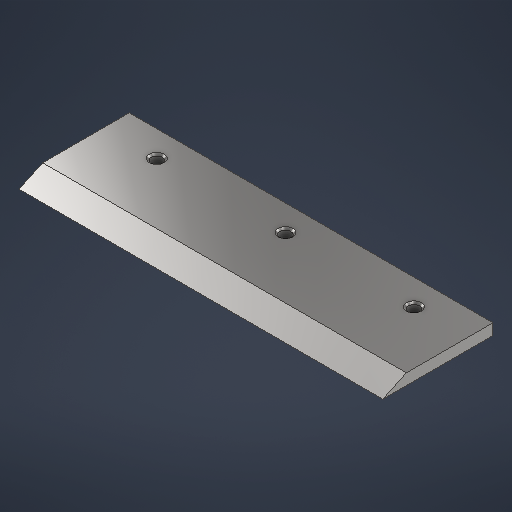
# Autodesk Inventor part: Knife
Saved by Autodesk Inventor 2027 (Build 310192000, 192)
## iProperties
Created: 2026-04-01
Part Number: Knife
Material: Ocel, uhlík
Document SubType Name: Modeling
Designer: zak
Density: 7.85 g/cm^3
Appearance: Pololeštěná
Author: zak
Autodesk Inventor part; units mm, degrees
ref_plane "YZ Plane" through (0, 0, 0) normal (1, 0, 0) x (0, 1, 0)
ref_plane "XZ Plane" through (0, 0, 0) normal (0, 1, 0) x (-1, 0, 0)
ref_plane "XY Plane" through (0, 0, 0) normal (0, 0, 1) x (1, 0, 0)
sketch "Náčrt1" plane through (0, 0, 0) normal (1, 0, 0) x (0, 1, 0)
  line L0 (1.5, 15) -> (-1.5, 15)
  line L1 (-1.5, 15) -> (-1.5, -15)
  line L2 (-1.5, -15) -> (1.5, -15)
  line L3 (1.5, -15) -> (1.5, 15)
  line L4 (1.5, 15) -> (-1.5, -15) construction
  line L5 (-1.5, 15) -> (1.5, -15) construction
  line L6 (-1.5, 15) -> (1.5, 8.5665)
  point P0 (0, 0)
  dimension "d0" = 3
  dimension "d1" = 30
  dimension "d2" = 25
  constraints: 14 end point, 2 midpoint, 2 parallel, 1 horizontal, 1 perpendicular, 1 point on line
  measures "d0" distance between parallel lines of L1 L3
  measures "d1" distance between parallel lines of L0 L2
  measures "d2" angle of L1 L6
extrude "Vysunutí1" add sketch "Náčrt1" along normal mid plane 99 contours L6 L3 L2 L1
sketch "Náčrt2" plane through (-49.5, -1.5, -15) normal (0, -1, 0) x (1, 0, 0)
  circle A0 centre (84.5, 7) radius 1.5
  circle A1 centre (49.5, 7) radius 1.5
  circle A2 centre (14.5, 7) radius 1.5
  line L0 (0, 0) -> (99, 0) projected
  line L1 (99, 30) -> (99, 0) projected
  line L2 (0, 30) -> (99, 30) projected
  line L3 (0, 0) -> (0, 30) projected
  line L4 (99, 7) -> (0, 7) construction
  line L5 (49.5, 0) -> (49.5, 30) construction
  point P0 (49.5, 15)
  dimension "d5" = 7
  dimension "d6" = 3
  dimension "d7" = 35
  dimension "d8" = 3
  constraints: 4 end point, 4 point on line, 3 centre point, 3 midpoint, 1 coincident, 1 perpendicular, 1 other
  measures "d5" distance between parallel lines of L0 L4
  measures "d6" diameter of A1
  measures "d7" distance of A1.centre A2.centre
  measures "d8" diameter of A2
extrude "Vysunutí2" cut sketch "Náčrt2" against normal through all contours A0 | A1 | A2
thread "Závit1" size "M3x0.5" class "6H" standard "ANSI Metric M Profile" full length
thread "Závit2" size "M3x0.5" class "6H" standard "ANSI Metric M Profile" full length
thread "Závit3" size "M3x0.5" class "6H" standard "ANSI Metric M Profile" full length
sketch "Náčrt3" plane through (-49.5, -1.5, -15) normal (0, -1, 0) x (1, 0, 0)
  circle A0 centre (14.5, 7) radius 1.5 projected
  circle A1 centre (49.5, 7) radius 1.5 projected
  circle A2 centre (84.5, 7) radius 1.5 projected
  line L0 (0, 0) -> (99, 0) projected
  line L1 (99, 30) -> (99, 0) projected
  line L2 (0, 30) -> (99, 30) projected
  line L3 (0, 0) -> (0, 30) projected
  line L4 (98.5, 0.5) -> (53.2335, 0.5) construction
  line L5 (53.2335, 0.5) -> (53.2335, 9.4631) construction
  line L6 (53.2335, 9.4631) -> (98.5, 9.4631) construction
  line L7 (98.5, 9.4631) -> (98.5, 0.5) construction
  line L8 (97.4789, 1.7723) -> (97.6653, 1.7723)
  line L9 (97.6653, 1.7723) -> (98.2184, 0.6945)
  line L10 (98.2184, 0.6945) -> (98.2184, 1.7723)
  line L11 (98.2184, 1.7723) -> (98.3734, 1.7723)
  line L12 (98.3734, 1.7723) -> (98.3734, 0.5223)
  line L13 (98.3734, 0.5223) -> (98.1374, 0.5223)
  line L14 (98.1374, 0.5223) -> (97.6339, 1.512)
  line L15 (97.6339, 1.512) -> (97.6339, 0.5223)
  line L16 (97.6339, 0.5223) -> (97.4789, 0.5223)
  line L17 (97.4789, 0.5223) -> (97.4789, 1.7723)
  spline S0 degree 2 poles (96.8306, 1.7936) (97.0555, 1.7936) (97.3027, 1.5413) (97.3027, 1.3083) knots 0 0 0 1 2 2 2
  spline S1 degree 2 poles (97.3027, 1.3083) (97.3027, 1.0794) (97.0626, 0.8079) (96.8691, 0.8079) knots 0 0 0 1 2 2 2
  spline S2 degree 2 poles (96.8691, 0.8079) (96.782, 0.8079) (96.6473, 0.8586) (96.5976, 0.9123) knots 0 0 0 1 2 2 2
  spline S3 degree 2 poles (96.5976, 0.9123) (96.547, 0.966) (96.4933, 1.1209) (96.4933, 1.2334) knots 0 0 0 1 2 2 2
  line L18 (96.4933, 1.2334) -> (96.4933, 1.3195)
  line L19 (96.4933, 1.3195) -> (97.1426, 1.3195)
  spline S4 degree 2 poles (97.1426, 1.3195) (97.1426, 1.4826) (96.9785, 1.6558) (96.8327, 1.6558) knots 0 0 0 1 2 2 2
  spline S5 degree 2 poles (96.8327, 1.6558) (96.781, 1.6558) (96.6807, 1.6325) (96.6402, 1.6143) knots 0 0 0 1 2 2 2
  spline S6 degree 2 poles (96.6402, 1.6143) (96.5976, 1.594) (96.5389, 1.5585) (96.5197, 1.5423) knots 0 0 0 1 2 2 2
  line L20 (96.5197, 1.5423) -> (96.5105, 1.5423)
  line L21 (96.5105, 1.5423) -> (96.5105, 1.7145)
  spline S7 degree 2 poles (96.5105, 1.7145) (96.5379, 1.7257) (96.6209, 1.7581) (96.6534, 1.7672) knots 0 0 0 1 2 2 2
  spline S8 degree 2 poles (96.6534, 1.7672) (96.6989, 1.7804) (96.7739, 1.7936) (96.8306, 1.7936) knots 0 0 0 1 2 2 2
  spline S9 degree 2 poles (96.6473, 1.1989) (96.6493, 1.1351) (96.6756, 1.0419) (96.701, 1.0105) knots 0 0 0 1 2 2 2
  spline S10 degree 2 poles (96.701, 1.0105) (96.7283, 0.9751) (96.8144, 0.9376) (96.8782, 0.9376) knots 0 0 0 1 2 2 2
  spline S11 degree 2 poles (96.8782, 0.9376) (96.941, 0.9376) (97.0292, 0.9751) (97.0656, 1.0115) knots 0 0 0 1 2 2 2
  spline S12 degree 2 poles (97.0656, 1.0115) (97.1011, 1.049) (97.1376, 1.1392) (97.1426, 1.1989) knots 0 0 0 1 2 2 2
  line L22 (97.1426, 1.1989) -> (96.6473, 1.1989)
  spline S13 degree 2 poles (95.5624, 1.3033) (95.5624, 1.5403) (95.7903, 1.7986) (95.9808, 1.7986) knots 0 0 0 1 2 2 2
  spline S14 degree 2 poles (95.9808, 1.7986) (96.1763, 1.7986) (96.4001, 1.5322) (96.4001, 1.3033) knots 0 0 0 1 2 2 2
  spline S15 degree 2 poles (96.4001, 1.3033) (96.4001, 1.0683) (96.1692, 0.8079) (95.9808, 0.8079) knots 0 0 0 1 2 2 2
  spline S16 degree 2 poles (95.9808, 0.8079) (95.7903, 0.8079) (95.5624, 1.0673) (95.5624, 1.3033) knots 0 0 0 1 2 2 2
  spline S17 degree 2 poles (95.7255, 1.3033) (95.7255, 1.1209) (95.8582, 0.9437) (95.9808, 0.9437) knots 0 0 0 1 2 2 2
  spline S18 degree 2 poles (95.9808, 0.9437) (96.1033, 0.9437) (96.237, 1.1209) (96.237, 1.3033) knots 0 0 0 1 2 2 2
  spline S19 degree 2 poles (96.237, 1.3033) (96.237, 1.4806) (96.1033, 1.6629) (95.9808, 1.6629) knots 0 0 0 1 2 2 2
  spline S20 degree 2 poles (95.9808, 1.6629) (95.8592, 1.6629) (95.7255, 1.4836) (95.7255, 1.3033) knots 0 0 0 1 2 2 2
  spline S21 degree 2 poles (95.0397, 1.7946) (95.1754, 1.7946) (95.3659, 1.7378) (95.45, 1.6973) knots 0 0 0 1 2 2 2
  line L23 (95.45, 1.6973) -> (95.45, 1.4887)
  line L24 (95.45, 1.4887) -> (95.4378, 1.4887)
  spline S22 degree 2 poles (95.4378, 1.4887) (95.3558, 1.5656) (95.1481, 1.6507) (95.0519, 1.6507) knots 0 0 0 1 2 2 2
  spline S23 degree 2 poles (95.0519, 1.6507) (94.9141, 1.6507) (94.7733, 1.5363) (94.7733, 1.4421) knots 0 0 0 1 2 2 2
  spline S24 degree 2 poles (94.7733, 1.4421) (94.7733, 1.3671) (94.8472, 1.2739) (94.9273, 1.2506) knots 0 0 0 1 2 2 2
  spline S25 degree 2 poles (94.9273, 1.2506) (94.985, 1.2344) (95.0812, 1.2121) (95.1532, 1.1939) knots 0 0 0 1 2 2 2
  spline S26 degree 2 poles (95.1532, 1.1939) (95.218, 1.1767) (95.3203, 1.125) (95.3598, 1.0835) knots 0 0 0 1 2 2 2
  spline S27 degree 2 poles (95.3598, 1.0835) (95.3983, 1.0419) (95.4408, 0.9305) (95.4408, 0.8576) knots 0 0 0 1 2 2 2
  spline S28 degree 2 poles (95.4408, 0.8576) (95.4408, 0.7056) (95.2038, 0.5) (95.0205, 0.5) knots 0 0 0 1 2 2 2
  spline S29 degree 2 poles (95.0205, 0.5) (94.9151, 0.5) (94.7287, 0.5415) (94.6487, 0.581) knots 0 0 0 1 2 2 2
  line L25 (94.6487, 0.581) -> (94.6487, 0.7796)
  line L26 (94.6487, 0.7796) -> (94.6609, 0.7796)
  spline S30 degree 2 poles (94.6609, 0.7796) (94.7206, 0.7249) (94.907, 0.6438) (95.0093, 0.6438) knots 0 0 0 1 2 2 2
  spline S31 degree 2 poles (95.0093, 0.6438) (95.1248, 0.6438) (95.2676, 0.7522) (95.2676, 0.8404) knots 0 0 0 1 2 2 2
  spline S32 degree 2 poles (95.2676, 0.8404) (95.2676, 0.9194) (95.1835, 1.0136) (95.1045, 1.0348) knots 0 0 0 1 2 2 2
  spline S33 degree 2 poles (95.1045, 1.0348) (95.0519, 1.049) (94.8989, 1.0855) (94.8483, 1.1007) knots 0 0 0 1 2 2 2
  spline S34 degree 2 poles (94.8483, 1.1007) (94.7196, 1.1402) (94.6001, 1.2992) (94.6001, 1.4157) knots 0 0 0 1 2 2 2
  spline S35 degree 2 poles (94.6001, 1.4157) (94.6001, 1.4897) (94.6598, 1.6315) (94.7135, 1.6811) knots 0 0 0 1 2 2 2
  spline S36 degree 2 poles (94.7135, 1.6811) (94.7733, 1.7358) (94.9252, 1.7946) (95.0397, 1.7946) knots 0 0 0 1 2 2 2
  line L27 (93.7137, 1.7723) -> (93.8718, 1.7723)
  line L28 (93.8718, 1.7723) -> (93.8718, 1.669)
  spline S37 degree 2 poles (93.8718, 1.669) (93.9447, 1.7328) (94.0754, 1.7986) (94.1564, 1.7986) knots 0 0 0 1 2 2 2
  spline S38 degree 2 poles (94.1564, 1.7986) (94.2172, 1.7986) (94.3256, 1.7581) (94.3651, 1.7145) knots 0 0 0 1 2 2 2
  spline S39 degree 2 poles (94.3651, 1.7145) (94.4056, 1.671) (94.4502, 1.5383) (94.4502, 1.4431) knots 0 0 0 1 2 2 2
  line L29 (94.4502, 1.4431) -> (94.4502, 0.8343)
  line L30 (94.4502, 0.8343) -> (94.2921, 0.8343)
  line L31 (94.2921, 0.8343) -> (94.2921, 1.3691)
  spline S40 degree 2 poles (94.2921, 1.3691) (94.2921, 1.4441) (94.281, 1.5423) (94.2618, 1.5788) knots 0 0 0 1 2 2 2
  spline S41 degree 2 poles (94.2618, 1.5788) (94.2425, 1.6153) (94.1767, 1.6487) (94.1149, 1.6487) knots 0 0 0 1 2 2 2
  spline S42 degree 2 poles (94.1149, 1.6487) (94.0571, 1.6487) (93.9265, 1.5829) (93.8718, 1.5353) knots 0 0 0 1 2 2 2
  line L32 (93.8718, 1.5353) -> (93.8718, 0.8343)
  line L33 (93.8718, 0.8343) -> (93.7137, 0.8343)
  line L34 (93.7137, 0.8343) -> (93.7137, 1.7723)
  line L35 (92.4212, 1.7723) -> (92.4212, 1.2293)
  spline S43 degree 2 poles (92.4212, 1.2293) (92.4212, 1.1645) (92.4313, 1.0541) (92.4475, 1.0237) knots 0 0 0 1 2 2 2
  spline S44 degree 2 poles (92.4475, 1.0237) (92.4637, 0.9903) (92.5255, 0.9579) (92.5792, 0.9579) knots 0 0 0 1 2 2 2
  spline S45 degree 2 poles (92.5792, 0.9579) (92.6278, 0.9579) (92.7393, 1.0176) (92.798, 1.0744) knots 0 0 0 1 2 2 2
  spline S46 degree 2 poles (92.798, 1.0744) (92.797, 1.0885) (92.795, 1.128) (92.795, 1.1544) knots 0 0 0 1 2 2 2
  line L36 (92.795, 1.1544) -> (92.795, 1.7723)
  line L37 (92.795, 1.7723) -> (92.953, 1.7723)
  line L38 (92.953, 1.7723) -> (92.953, 1.2293)
  spline S47 degree 2 poles (92.953, 1.2293) (92.953, 1.1645) (92.9631, 1.0541) (92.9793, 1.0237) knots 0 0 0 1 2 2 2
  spline S48 degree 2 poles (92.9793, 1.0237) (92.9955, 0.9903) (93.0573, 0.9579) (93.111, 0.9579) knots 0 0 0 1 2 2 2
  spline S49 degree 2 poles (93.111, 0.9579) (93.1617, 0.9579) (93.2741, 1.0217) (93.3268, 1.0713) knots 0 0 0 1 2 2 2
  line L39 (93.3268, 1.0713) -> (93.3268, 1.7723)
  line L40 (93.3268, 1.7723) -> (93.4848, 1.7723)
  line L41 (93.4848, 1.7723) -> (93.4848, 0.8343)
  line L42 (93.4848, 0.8343) -> (93.3268, 0.8343)
  line L43 (93.3268, 0.8343) -> (93.3268, 0.9376)
  spline S50 degree 2 poles (93.3268, 0.9376) (93.265, 0.8758) (93.1434, 0.8079) (93.0705, 0.8079) knots 0 0 0 1 2 2 2
  spline S51 degree 2 poles (93.0705, 0.8079) (92.9874, 0.8079) (92.8588, 0.8839) (92.8254, 0.97) knots 0 0 0 1 2 2 2
  spline S52 degree 2 poles (92.8254, 0.97) (92.7534, 0.89) (92.6177, 0.8079) (92.5387, 0.8079) knots 0 0 0 1 2 2 2
  spline S53 degree 2 poles (92.5387, 0.8079) (92.4779, 0.8079) (92.3786, 0.8454) (92.3422, 0.888) knots 0 0 0 1 2 2 2
  spline S54 degree 2 poles (92.3422, 0.888) (92.3047, 0.9305) (92.2632, 1.0581) (92.2632, 1.1544) knots 0 0 0 1 2 2 2
  line L44 (92.2632, 1.1544) -> (92.2632, 1.7723)
  line L45 (92.2632, 1.7723) -> (92.4212, 1.7723)
  spline S55 degree 2 poles (91.6341, 1.7936) (91.859, 1.7936) (92.1062, 1.5413) (92.1062, 1.3083) knots 0 0 0 1 2 2 2
  spline S56 degree 2 poles (92.1062, 1.3083) (92.1062, 1.0794) (91.8661, 0.8079) (91.6726, 0.8079) knots 0 0 0 1 2 2 2
  spline S57 degree 2 poles (91.6726, 0.8079) (91.5855, 0.8079) (91.4508, 0.8586) (91.4011, 0.9123) knots 0 0 0 1 2 2 2
  spline S58 degree 2 poles (91.4011, 0.9123) (91.3505, 0.966) (91.2968, 1.1209) (91.2968, 1.2334) knots 0 0 0 1 2 2 2
  line L46 (91.2968, 1.2334) -> (91.2968, 1.3195)
  line L47 (91.2968, 1.3195) -> (91.9461, 1.3195)
  spline S59 degree 2 poles (91.9461, 1.3195) (91.9461, 1.4826) (91.782, 1.6558) (91.6361, 1.6558) knots 0 0 0 1 2 2 2
  spline S60 degree 2 poles (91.6361, 1.6558) (91.5845, 1.6558) (91.4842, 1.6325) (91.4437, 1.6143) knots 0 0 0 1 2 2 2
  spline S61 degree 2 poles (91.4437, 1.6143) (91.4011, 1.594) (91.3424, 1.5585) (91.3231, 1.5423) knots 0 0 0 1 2 2 2
  line L48 (91.3231, 1.5423) -> (91.314, 1.5423)
  line L49 (91.314, 1.5423) -> (91.314, 1.7145)
  spline S62 degree 2 poles (91.314, 1.7145) (91.3414, 1.7257) (91.4244, 1.7581) (91.4568, 1.7672) knots 0 0 0 1 2 2 2
  spline S63 degree 2 poles (91.4568, 1.7672) (91.5024, 1.7804) (91.5774, 1.7936) (91.6341, 1.7936) knots 0 0 0 1 2 2 2
  spline S64 degree 2 poles (91.4508, 1.1989) (91.4528, 1.1351) (91.4791, 1.0419) (91.5045, 1.0105) knots 0 0 0 1 2 2 2
  spline S65 degree 2 poles (91.5045, 1.0105) (91.5318, 0.9751) (91.6179, 0.9376) (91.6817, 0.9376) knots 0 0 0 1 2 2 2
  spline S66 degree 2 poles (91.6817, 0.9376) (91.7445, 0.9376) (91.8327, 0.9751) (91.8691, 1.0115) knots 0 0 0 1 2 2 2
  spline S67 degree 2 poles (91.8691, 1.0115) (91.9046, 1.049) (91.941, 1.1392) (91.9461, 1.1989) knots 0 0 0 1 2 2 2
  line L50 (91.9461, 1.1989) -> (91.4508, 1.1989)
  spline S68 degree 2 poles (90.764, 1.7936) (90.8612, 1.7936) (91.0223, 1.7338) (91.08, 1.673) knots 0 0 0 1 2 2 2
  spline S69 degree 2 poles (91.08, 1.673) (91.1378, 1.6132) (91.2016, 1.4289) (91.2016, 1.3053) knots 0 0 0 1 2 2 2
  spline S70 degree 2 poles (91.2016, 1.3053) (91.2016, 1.1817) (91.1357, 1.0014) (91.08, 0.9406) knots 0 0 0 1 2 2 2
  spline S71 degree 2 poles (91.08, 0.9406) (91.0243, 0.8788) (90.8592, 0.813) (90.764, 0.813) knots 0 0 0 1 2 2 2
  spline S72 degree 2 poles (90.764, 0.813) (90.687, 0.813) (90.5432, 0.8566) (90.4874, 0.8849) knots 0 0 0 1 2 2 2
  line L51 (90.4874, 0.8849) -> (90.4874, 1.0622)
  line L52 (90.4874, 1.0622) -> (90.4966, 1.0622)
  spline S73 degree 2 poles (90.4966, 1.0622) (90.5138, 1.048) (90.5665, 1.0115) (90.6039, 0.9923) knots 0 0 0 1 2 2 2
  spline S74 degree 2 poles (90.6039, 0.9923) (90.6374, 0.9761) (90.7265, 0.9508) (90.767, 0.9508) knots 0 0 0 1 2 2 2
  spline S75 degree 2 poles (90.767, 0.9508) (90.8896, 0.9508) (91.0385, 1.1361) (91.0385, 1.3053) knots 0 0 0 1 2 2 2
  spline S76 degree 2 poles (91.0385, 1.3053) (91.0385, 1.4704) (90.8947, 1.6558) (90.767, 1.6558) knots 0 0 0 1 2 2 2
  spline S77 degree 2 poles (90.767, 1.6558) (90.69, 1.6558) (90.5502, 1.592) (90.4966, 1.5423) knots 0 0 0 1 2 2 2
  line L53 (90.4966, 1.5423) -> (90.4874, 1.5423)
  line L54 (90.4874, 1.5423) -> (90.4874, 1.7196)
  spline S78 degree 2 poles (90.4874, 1.7196) (90.5107, 1.7308) (90.5816, 1.7622) (90.61, 1.7692) knots 0 0 0 1 2 2 2
  spline S79 degree 2 poles (90.61, 1.7692) (90.6505, 1.7814) (90.7143, 1.7936) (90.764, 1.7936) knots 0 0 0 1 2 2 2
  line L55 (89.3722, 1.3013) -> (89.8452, 1.3013)
  line L56 (89.8452, 1.3013) -> (89.8452, 1.1493)
  line L57 (89.8452, 1.1493) -> (89.3722, 1.1493)
  line L58 (89.3722, 1.1493) -> (89.3722, 1.3013)
  line L59 (87.562, 1.7723) -> (87.7281, 1.7723)
  line L60 (87.7281, 1.7723) -> (87.7281, 0.6955)
  line L61 (87.7281, 0.6955) -> (88.0543, 1.4279)
  line L62 (88.0543, 1.4279) -> (88.1556, 1.4279)
  line L63 (88.1556, 1.4279) -> (88.4787, 0.6955)
  line L64 (88.4787, 0.6955) -> (88.4787, 1.7723)
  line L65 (88.4787, 1.7723) -> (88.6337, 1.7723)
  line L66 (88.6337, 1.7723) -> (88.6337, 0.5223)
  line L67 (88.6337, 0.5223) -> (88.4068, 0.5223)
  line L68 (88.4068, 0.5223) -> (88.0948, 1.2182)
  line L69 (88.0948, 1.2182) -> (87.7929, 0.5223)
  line L70 (87.7929, 0.5223) -> (87.562, 0.5223)
  line L71 (87.562, 0.5223) -> (87.562, 1.7723)
  line L72 (86.3971, 1.7723) -> (86.6128, 1.7723)
  line L73 (86.6128, 1.7723) -> (87.0697, 1.1908)
  line L74 (87.0697, 1.1908) -> (87.1426, 1.2729)
  line L75 (87.1426, 1.2729) -> (87.1426, 1.7723)
  line L76 (87.1426, 1.7723) -> (87.3088, 1.7723)
  line L77 (87.3088, 1.7723) -> (87.3088, 0.5223)
  line L78 (87.3088, 0.5223) -> (87.1426, 0.5223)
  line L79 (87.1426, 0.5223) -> (87.1426, 1.0966)
  line L80 (87.1426, 1.0966) -> (86.6301, 0.5223)
  line L81 (86.6301, 0.5223) -> (86.4275, 0.5223)
  line L82 (86.4275, 0.5223) -> (86.9451, 1.0804)
  line L83 (86.9451, 1.0804) -> (86.3971, 1.7723)
  line L84 (85.6252, 1.7723) -> (86.235, 1.7723)
  line L85 (86.235, 1.7723) -> (86.235, 1.6447)
  line L86 (86.235, 1.6447) -> (86.0081, 1.6447)
  line L87 (86.0081, 1.6447) -> (86.0081, 0.8069)
  line L88 (86.0081, 0.8069) -> (86.235, 0.8069)
  line L89 (86.235, 0.8069) -> (86.235, 0.6925)
  spline S80 degree 2 poles (86.235, 0.6925) (86.1064, 0.6925) (85.9848, 0.6195) (85.9767, 0.5182) knots 0 0 0 1 2 2 2
  line L90 (85.9767, 0.5182) -> (85.847, 0.5182)
  line L91 (85.847, 0.5182) -> (85.847, 1.6447)
  line L92 (85.847, 1.6447) -> (85.6252, 1.6447)
  line L93 (85.6252, 1.6447) -> (85.6252, 1.7723)
  line L94 (97.3017, 3.8304) -> (97.4678, 3.8304)
  line L95 (97.4678, 3.8304) -> (97.4678, 2.7536)
  line L96 (97.4678, 2.7536) -> (97.794, 3.486)
  line L97 (97.794, 3.486) -> (97.8953, 3.486)
  line L98 (97.8953, 3.486) -> (98.2184, 2.7536)
  line L99 (98.2184, 2.7536) -> (98.2184, 3.8304)
  line L100 (98.2184, 3.8304) -> (98.3734, 3.8304)
  line L101 (98.3734, 3.8304) -> (98.3734, 2.5804)
  line L102 (98.3734, 2.5804) -> (98.1465, 2.5804)
  line L103 (98.1465, 2.5804) -> (97.8345, 3.2763)
  line L104 (97.8345, 3.2763) -> (97.5326, 2.5804)
  line L105 (97.5326, 2.5804) -> (97.3017, 2.5804)
  line L106 (97.3017, 2.5804) -> (97.3017, 3.8304)
  spline S81 degree 2 poles (96.5379, 3.7311) (96.5571, 3.7453) (96.622, 3.7959) (96.6524, 3.8111) knots 0 0 0 1 2 2 2
  spline S82 degree 2 poles (96.6524, 3.8111) (96.6939, 3.8334) (96.7719, 3.8567) (96.8428, 3.8567) knots 0 0 0 1 2 2 2
  spline S83 degree 2 poles (96.8428, 3.8567) (96.9005, 3.8567) (97.0049, 3.8132) (97.0444, 3.7737) knots 0 0 0 1 2 2 2
  spline S84 degree 2 poles (97.0444, 3.7737) (97.0818, 3.7352) (97.1274, 3.6217) (97.1274, 3.5589) knots 0 0 0 1 2 2 2
  spline S85 degree 2 poles (97.1274, 3.5589) (97.1274, 3.4617) (97.0454, 3.3239) (96.9562, 3.2844) knots 0 0 0 1 2 2 2
  spline S86 degree 2 poles (96.9562, 3.2844) (96.8772, 3.2479) (96.6625, 3.2206) (96.5379, 3.2135) knots 0 0 0 1 2 2 2
  line L107 (96.5379, 3.2135) -> (96.5379, 3.1831)
  spline S87 degree 2 poles (96.5379, 3.1831) (96.5379, 3.1284) (96.5713, 3.0605) (96.6017, 3.0413) knots 0 0 0 1 2 2 2
  spline S88 degree 2 poles (96.6017, 3.0413) (96.6321, 3.022) (96.7192, 3.0099) (96.7658, 3.0099) knots 0 0 0 1 2 2 2
  spline S89 degree 2 poles (96.7658, 3.0099) (96.8205, 3.0099) (96.9684, 3.0423) (97.0423, 3.0737) knots 0 0 0 1 2 2 2
  line L108 (97.0423, 3.0737) -> (97.0515, 3.0737)
  line L109 (97.0515, 3.0737) -> (97.0515, 2.9126)
  spline S90 degree 2 poles (97.0515, 2.9126) (97.0079, 2.9005) (96.8448, 2.8701) (96.7648, 2.8701) knots 0 0 0 1 2 2 2
  spline S91 degree 2 poles (96.7648, 2.8701) (96.6675, 2.8701) (96.5348, 2.9005) (96.4822, 2.94) knots 0 0 0 1 2 2 2
  spline S92 degree 2 poles (96.4822, 2.94) (96.4305, 2.9785) (96.3799, 3.101) (96.3799, 3.1892) knots 0 0 0 1 2 2 2
  line L110 (96.3799, 3.1892) -> (96.3799, 3.8304)
  line L111 (96.3799, 3.8304) -> (96.5379, 3.8304)
  line L112 (96.5379, 3.8304) -> (96.5379, 3.7311)
  line L113 (96.5379, 3.5994) -> (96.5379, 3.3391)
  spline S93 degree 2 poles (96.5379, 3.3391) (96.5946, 3.3442) (96.7658, 3.3614) (96.8195, 3.3776) knots 0 0 0 1 2 2 2
  spline S94 degree 2 poles (96.8195, 3.3776) (96.8823, 3.3968) (96.9643, 3.4769) (96.9643, 3.5478) knots 0 0 0 1 2 2 2
  spline S95 degree 2 poles (96.9643, 3.5478) (96.9643, 3.6288) (96.8732, 3.7108) (96.7861, 3.7108) knots 0 0 0 1 2 2 2
  spline S96 degree 2 poles (96.7861, 3.7108) (96.7121, 3.7108) (96.5906, 3.647) (96.5379, 3.5994) knots 0 0 0 1 2 2 2
  line L114 (95.4368, 3.8304) -> (95.5948, 3.8304)
  line L115 (95.5948, 3.8304) -> (95.5948, 3.7352)
  spline S97 degree 2 poles (95.5948, 3.7352) (95.6313, 3.7655) (95.685, 3.8061) (95.7214, 3.8233) knots 0 0 0 1 2 2 2
  spline S98 degree 2 poles (95.7214, 3.8233) (95.7549, 3.8395) (95.8268, 3.8567) (95.8744, 3.8567) knots 0 0 0 1 2 2 2
  spline S99 degree 2 poles (95.8744, 3.8567) (95.9514, 3.8567) (96.081, 3.7929) (96.1266, 3.7311) knots 0 0 0 1 2 2 2
  spline S100 degree 2 poles (96.1266, 3.7311) (96.1722, 3.6693) (96.2229, 3.487) (96.2229, 3.3685) knots 0 0 0 1 2 2 2
  spline S101 degree 2 poles (96.2229, 3.3685) (96.2229, 3.2449) (96.159, 3.0646) (96.1033, 2.9967) knots 0 0 0 1 2 2 2
  spline S102 degree 2 poles (96.1033, 2.9967) (96.0517, 2.9359) (95.9068, 2.866) (95.8268, 2.866) knots 0 0 0 1 2 2 2
  spline S103 degree 2 poles (95.8268, 2.866) (95.7569, 2.866) (95.6526, 2.8974) (95.5948, 2.9299) knots 0 0 0 1 2 2 2
  line L116 (95.5948, 2.9299) -> (95.5948, 2.5247)
  line L117 (95.5948, 2.5247) -> (95.4368, 2.5247)
  line L118 (95.4368, 2.5247) -> (95.4368, 3.8304)
  line L119 (95.5948, 3.6025) -> (95.5948, 3.0605)
  spline S104 degree 2 poles (95.5948, 3.0605) (95.6536, 3.0322) (95.7468, 3.0109) (95.8004, 3.0109) knots 0 0 0 1 2 2 2
  spline S105 degree 2 poles (95.8004, 3.0109) (95.922, 3.0109) (96.0598, 3.1932) (96.0598, 3.3654) knots 0 0 0 1 2 2 2
  spline S106 degree 2 poles (96.0598, 3.3654) (96.0598, 3.5316) (95.9544, 3.7068) (95.8379, 3.7068) knots 0 0 0 1 2 2 2
  spline S107 degree 2 poles (95.8379, 3.7068) (95.7761, 3.7068) (95.6505, 3.6501) (95.5948, 3.6025) knots 0 0 0 1 2 2 2
  spline S108 degree 2 poles (94.8006, 3.8516) (95.0255, 3.8516) (95.2727, 3.5994) (95.2727, 3.3664) knots 0 0 0 1 2 2 2
  spline S109 degree 2 poles (95.2727, 3.3664) (95.2727, 3.1375) (95.0326, 2.866) (94.8391, 2.866) knots 0 0 0 1 2 2 2
  spline S110 degree 2 poles (94.8391, 2.866) (94.752, 2.866) (94.6173, 2.9167) (94.5677, 2.9704) knots 0 0 0 1 2 2 2
  spline S111 degree 2 poles (94.5677, 2.9704) (94.517, 3.0241) (94.4633, 3.179) (94.4633, 3.2915) knots 0 0 0 1 2 2 2
  line L120 (94.4633, 3.2915) -> (94.4633, 3.3776)
  line L121 (94.4633, 3.3776) -> (95.1126, 3.3776)
  spline S112 degree 2 poles (95.1126, 3.3776) (95.1126, 3.5407) (94.9485, 3.7139) (94.8027, 3.7139) knots 0 0 0 1 2 2 2
  spline S113 degree 2 poles (94.8027, 3.7139) (94.751, 3.7139) (94.6507, 3.6906) (94.6102, 3.6724) knots 0 0 0 1 2 2 2
  spline S114 degree 2 poles (94.6102, 3.6724) (94.5677, 3.6521) (94.5089, 3.6166) (94.4897, 3.6004) knots 0 0 0 1 2 2 2
  line L122 (94.4897, 3.6004) -> (94.4806, 3.6004)
  line L123 (94.4806, 3.6004) -> (94.4806, 3.7726)
  spline S115 degree 2 poles (94.4806, 3.7726) (94.5079, 3.7838) (94.591, 3.8162) (94.6234, 3.8253) knots 0 0 0 1 2 2 2
  spline S116 degree 2 poles (94.6234, 3.8253) (94.669, 3.8385) (94.7439, 3.8516) (94.8006, 3.8516) knots 0 0 0 1 2 2 2
  spline S117 degree 2 poles (94.6173, 3.257) (94.6193, 3.1932) (94.6457, 3.1) (94.671, 3.0686) knots 0 0 0 1 2 2 2
  spline S118 degree 2 poles (94.671, 3.0686) (94.6983, 3.0332) (94.7844, 2.9957) (94.8483, 2.9957) knots 0 0 0 1 2 2 2
  spline S119 degree 2 poles (94.8483, 2.9957) (94.9111, 2.9957) (94.9992, 3.0332) (95.0357, 3.0696) knots 0 0 0 1 2 2 2
  spline S120 degree 2 poles (95.0357, 3.0696) (95.0711, 3.1071) (95.1076, 3.1973) (95.1126, 3.257) knots 0 0 0 1 2 2 2
  line L124 (95.1126, 3.257) -> (94.6173, 3.257)
  spline S121 degree 2 poles (92.9803, 3.3462) (92.9803, 3.5761) (93.2032, 3.8567) (93.3714, 3.8567) knots 0 0 0 1 2 2 2
  spline S122 degree 2 poles (93.3714, 3.8567) (93.4473, 3.8567) (93.5557, 3.8192) (93.6084, 3.7868) knots 0 0 0 1 2 2 2
  line L125 (93.6084, 3.7868) -> (93.6185, 3.8304)
  line L126 (93.6185, 3.8304) -> (93.7664, 3.8304)
  line L127 (93.7664, 3.8304) -> (93.7664, 2.5247)
  line L128 (93.7664, 2.5247) -> (93.6084, 2.5247)
  line L129 (93.6084, 2.5247) -> (93.6084, 2.9906)
  spline S123 degree 2 poles (93.6084, 2.9906) (93.5486, 2.9369) (93.4098, 2.866) (93.3217, 2.866) knots 0 0 0 1 2 2 2
  spline S124 degree 2 poles (93.3217, 2.866) (93.1627, 2.866) (92.9803, 3.1203) (92.9803, 3.3462) knots 0 0 0 1 2 2 2
  spline S125 degree 2 poles (93.1434, 3.3583) (93.1434, 3.1902) (93.2457, 3.016) (93.3592, 3.016) knots 0 0 0 1 2 2 2
  spline S126 degree 2 poles (93.3592, 3.016) (93.423, 3.016) (93.5547, 3.0767) (93.6084, 3.1233) knots 0 0 0 1 2 2 2
  line L130 (93.6084, 3.1233) -> (93.6084, 3.6612)
  spline S127 degree 2 poles (93.6084, 3.6612) (93.5486, 3.6906) (93.4564, 3.7149) (93.4017, 3.7149) knots 0 0 0 1 2 2 2
  spline S128 degree 2 poles (93.4017, 3.7149) (93.2812, 3.7149) (93.1434, 3.5437) (93.1434, 3.3583) knots 0 0 0 1 2 2 2
  line L131 (92.0798, 2.8924) -> (92.5843, 4.1758)
  line L132 (92.5843, 4.1758) -> (92.7534, 4.1758)
  line L133 (92.7534, 4.1758) -> (92.5853, 3.7848)
  line L134 (92.5853, 3.7848) -> (92.9256, 2.8924)
  line L135 (92.9256, 2.8924) -> (92.7555, 2.8924)
  line L136 (92.7555, 2.8924) -> (92.4992, 3.5873)
  line L137 (92.4992, 3.5873) -> (92.2439, 2.8924)
  line L138 (92.2439, 2.8924) -> (92.0798, 2.8924)
  line L139 (90.5047, 2.5804) -> (90.9352, 3.8304)
  line L140 (90.9352, 3.8304) -> (91.1145, 3.8304)
  line L141 (91.1145, 3.8304) -> (91.545, 2.5804)
  line L142 (91.545, 2.5804) -> (91.3667, 2.5804)
  line L143 (91.3667, 2.5804) -> (91.0203, 3.6187)
  line L144 (91.0203, 3.6187) -> (90.6738, 2.5804)
  line L145 (90.6738, 2.5804) -> (90.5047, 2.5804)
  spline S129 degree 2 poles (89.8746, 3.7311) (89.8938, 3.7453) (89.9587, 3.7959) (89.9891, 3.8111) knots 0 0 0 1 2 2 2
  spline S130 degree 2 poles (89.9891, 3.8111) (90.0306, 3.8334) (90.1086, 3.8567) (90.1795, 3.8567) knots 0 0 0 1 2 2 2
  spline S131 degree 2 poles (90.1795, 3.8567) (90.2372, 3.8567) (90.3416, 3.8132) (90.3811, 3.7737) knots 0 0 0 1 2 2 2
  spline S132 degree 2 poles (90.3811, 3.7737) (90.4186, 3.7352) (90.4641, 3.6217) (90.4641, 3.5589) knots 0 0 0 1 2 2 2
  spline S133 degree 2 poles (90.4641, 3.5589) (90.4641, 3.4617) (90.3821, 3.3239) (90.2929, 3.2844) knots 0 0 0 1 2 2 2
  spline S134 degree 2 poles (90.2929, 3.2844) (90.2139, 3.2479) (89.9992, 3.2206) (89.8746, 3.2135) knots 0 0 0 1 2 2 2
  line L146 (89.8746, 3.2135) -> (89.8746, 3.1831)
  spline S135 degree 2 poles (89.8746, 3.1831) (89.8746, 3.1284) (89.908, 3.0605) (89.9384, 3.0413) knots 0 0 0 1 2 2 2
  spline S136 degree 2 poles (89.9384, 3.0413) (89.9688, 3.022) (90.0559, 3.0099) (90.1025, 3.0099) knots 0 0 0 1 2 2 2
  spline S137 degree 2 poles (90.1025, 3.0099) (90.1572, 3.0099) (90.3051, 3.0423) (90.3791, 3.0737) knots 0 0 0 1 2 2 2
  line L147 (90.3791, 3.0737) -> (90.3882, 3.0737)
  line L148 (90.3882, 3.0737) -> (90.3882, 2.9126)
  spline S138 degree 2 poles (90.3882, 2.9126) (90.3446, 2.9005) (90.1815, 2.8701) (90.1015, 2.8701) knots 0 0 0 1 2 2 2
  spline S139 degree 2 poles (90.1015, 2.8701) (90.0043, 2.8701) (89.8716, 2.9005) (89.8189, 2.94) knots 0 0 0 1 2 2 2
  spline S140 degree 2 poles (89.8189, 2.94) (89.7672, 2.9785) (89.7166, 3.101) (89.7166, 3.1892) knots 0 0 0 1 2 2 2
  line L149 (89.7166, 3.1892) -> (89.7166, 3.8304)
  line L150 (89.7166, 3.8304) -> (89.8746, 3.8304)
  line L151 (89.8746, 3.8304) -> (89.8746, 3.7311)
  line L152 (89.8746, 3.5994) -> (89.8746, 3.3391)
  spline S141 degree 2 poles (89.8746, 3.3391) (89.9313, 3.3442) (90.1025, 3.3614) (90.1562, 3.3776) knots 0 0 0 1 2 2 2
  spline S142 degree 2 poles (90.1562, 3.3776) (90.219, 3.3968) (90.3011, 3.4769) (90.3011, 3.5478) knots 0 0 0 1 2 2 2
  spline S143 degree 2 poles (90.3011, 3.5478) (90.3011, 3.6288) (90.2099, 3.7108) (90.1228, 3.7108) knots 0 0 0 1 2 2 2
  spline S144 degree 2 poles (90.1228, 3.7108) (90.0488, 3.7108) (89.9273, 3.647) (89.8746, 3.5994) knots 0 0 0 1 2 2 2
  line L153 (88.7735, 3.8304) -> (88.9315, 3.8304)
  line L154 (88.9315, 3.8304) -> (88.9315, 3.7352)
  spline S145 degree 2 poles (88.9315, 3.7352) (88.968, 3.7655) (89.0217, 3.8061) (89.0581, 3.8233) knots 0 0 0 1 2 2 2
  spline S146 degree 2 poles (89.0581, 3.8233) (89.0916, 3.8395) (89.1635, 3.8567) (89.2111, 3.8567) knots 0 0 0 1 2 2 2
  spline S147 degree 2 poles (89.2111, 3.8567) (89.2881, 3.8567) (89.4177, 3.7929) (89.4633, 3.7311) knots 0 0 0 1 2 2 2
  spline S148 degree 2 poles (89.4633, 3.7311) (89.5089, 3.6693) (89.5596, 3.487) (89.5596, 3.3685) knots 0 0 0 1 2 2 2
  spline S149 degree 2 poles (89.5596, 3.3685) (89.5596, 3.2449) (89.4957, 3.0646) (89.44, 2.9967) knots 0 0 0 1 2 2 2
  spline S150 degree 2 poles (89.44, 2.9967) (89.3884, 2.9359) (89.2435, 2.866) (89.1635, 2.866) knots 0 0 0 1 2 2 2
  spline S151 degree 2 poles (89.1635, 2.866) (89.0936, 2.866) (88.9893, 2.8974) (88.9315, 2.9299) knots 0 0 0 1 2 2 2
  line L155 (88.9315, 2.9299) -> (88.9315, 2.5247)
  line L156 (88.9315, 2.5247) -> (88.7735, 2.5247)
  line L157 (88.7735, 2.5247) -> (88.7735, 3.8304)
  line L158 (88.9315, 3.6025) -> (88.9315, 3.0605)
  spline S152 degree 2 poles (88.9315, 3.0605) (88.9903, 3.0322) (89.0835, 3.0109) (89.1372, 3.0109) knots 0 0 0 1 2 2 2
  spline S153 degree 2 poles (89.1372, 3.0109) (89.2587, 3.0109) (89.3965, 3.1932) (89.3965, 3.3654) knots 0 0 0 1 2 2 2
  spline S154 degree 2 poles (89.3965, 3.3654) (89.3965, 3.5316) (89.2911, 3.7068) (89.1746, 3.7068) knots 0 0 0 1 2 2 2
  spline S155 degree 2 poles (89.1746, 3.7068) (89.1128, 3.7068) (88.9872, 3.6501) (88.9315, 3.6025) knots 0 0 0 1 2 2 2
  line L159 (88.3835, 3.8304) -> (88.5415, 3.8304)
  line L160 (88.5415, 3.8304) -> (88.5415, 2.8924)
  line L161 (88.5415, 2.8924) -> (88.3835, 2.8924)
  line L162 (88.3835, 2.8924) -> (88.3835, 3.8304)
  line L163 (88.3724, 2.7364) -> (88.5517, 2.7364)
  line L164 (88.5517, 2.7364) -> (88.5517, 2.5723)
  line L165 (88.5517, 2.5723) -> (88.3724, 2.5723)
  line L166 (88.3724, 2.5723) -> (88.3724, 2.7364)
  line L167 (87.0879, 3.8304) -> (87.0879, 3.2874)
  spline S156 degree 2 poles (87.0879, 3.2874) (87.0879, 3.2226) (87.0981, 3.1122) (87.1143, 3.0818) knots 0 0 0 1 2 2 2
  spline S157 degree 2 poles (87.1143, 3.0818) (87.1305, 3.0484) (87.1923, 3.016) (87.2459, 3.016) knots 0 0 0 1 2 2 2
  spline S158 degree 2 poles (87.2459, 3.016) (87.2946, 3.016) (87.406, 3.0757) (87.4647, 3.1324) knots 0 0 0 1 2 2 2
  spline S159 degree 2 poles (87.4647, 3.1324) (87.4637, 3.1466) (87.4617, 3.1861) (87.4617, 3.2125) knots 0 0 0 1 2 2 2
  line L168 (87.4617, 3.2125) -> (87.4617, 3.8304)
  line L169 (87.4617, 3.8304) -> (87.6197, 3.8304)
  line L170 (87.6197, 3.8304) -> (87.6197, 3.2874)
  spline S160 degree 2 poles (87.6197, 3.2874) (87.6197, 3.2226) (87.6299, 3.1122) (87.6461, 3.0818) knots 0 0 0 1 2 2 2
  spline S161 degree 2 poles (87.6461, 3.0818) (87.6623, 3.0484) (87.7241, 3.016) (87.7778, 3.016) knots 0 0 0 1 2 2 2
  spline S162 degree 2 poles (87.7778, 3.016) (87.8284, 3.016) (87.9408, 3.0798) (87.9935, 3.1294) knots 0 0 0 1 2 2 2
  line L171 (87.9935, 3.1294) -> (87.9935, 3.8304)
  line L172 (87.9935, 3.8304) -> (88.1515, 3.8304)
  line L173 (88.1515, 3.8304) -> (88.1515, 2.8924)
  line L174 (88.1515, 2.8924) -> (87.9935, 2.8924)
  line L175 (87.9935, 2.8924) -> (87.9935, 2.9957)
  spline S163 degree 2 poles (87.9935, 2.9957) (87.9317, 2.9339) (87.8102, 2.866) (87.7372, 2.866) knots 0 0 0 1 2 2 2
  spline S164 degree 2 poles (87.7372, 2.866) (87.6542, 2.866) (87.5255, 2.942) (87.4921, 3.0281) knots 0 0 0 1 2 2 2
  spline S165 degree 2 poles (87.4921, 3.0281) (87.4202, 2.9481) (87.2844, 2.866) (87.2054, 2.866) knots 0 0 0 1 2 2 2
  spline S166 degree 2 poles (87.2054, 2.866) (87.1447, 2.866) (87.0454, 2.9035) (87.0089, 2.9461) knots 0 0 0 1 2 2 2
  spline S167 degree 2 poles (87.0089, 2.9461) (86.9714, 2.9886) (86.9299, 3.1162) (86.9299, 3.2125) knots 0 0 0 1 2 2 2
  line L176 (86.9299, 3.2125) -> (86.9299, 3.8304)
  line L177 (86.9299, 3.8304) -> (87.0879, 3.8304)
  spline S168 degree 2 poles (85.8106, 3.8527) (85.9463, 3.8527) (86.1368, 3.7959) (86.2208, 3.7554) knots 0 0 0 1 2 2 2
  line L178 (86.2208, 3.7554) -> (86.2208, 3.5467)
  line L179 (86.2208, 3.5467) -> (86.2087, 3.5467)
  spline S169 degree 2 poles (86.2087, 3.5467) (86.1266, 3.6237) (85.919, 3.7088) (85.8227, 3.7088) knots 0 0 0 1 2 2 2
  spline S170 degree 2 poles (85.8227, 3.7088) (85.685, 3.7088) (85.5442, 3.5944) (85.5442, 3.5002) knots 0 0 0 1 2 2 2
  spline S171 degree 2 poles (85.5442, 3.5002) (85.5442, 3.4252) (85.6181, 3.332) (85.6981, 3.3087) knots 0 0 0 1 2 2 2
  spline S172 degree 2 poles (85.6981, 3.3087) (85.7559, 3.2925) (85.8521, 3.2702) (85.924, 3.252) knots 0 0 0 1 2 2 2
  spline S173 degree 2 poles (85.924, 3.252) (85.9889, 3.2348) (86.0912, 3.1831) (86.1307, 3.1416) knots 0 0 0 1 2 2 2
  spline S174 degree 2 poles (86.1307, 3.1416) (86.1692, 3.1) (86.2117, 2.9886) (86.2117, 2.9157) knots 0 0 0 1 2 2 2
  spline S175 degree 2 poles (86.2117, 2.9157) (86.2117, 2.7637) (85.9747, 2.5581) (85.7913, 2.5581) knots 0 0 0 1 2 2 2
  spline S176 degree 2 poles (85.7913, 2.5581) (85.686, 2.5581) (85.4996, 2.5996) (85.4196, 2.6391) knots 0 0 0 1 2 2 2
  line L180 (85.4196, 2.6391) -> (85.4196, 2.8377)
  line L181 (85.4196, 2.8377) -> (85.4317, 2.8377)
  spline S177 degree 2 poles (85.4317, 2.8377) (85.4915, 2.783) (85.6779, 2.7019) (85.7802, 2.7019) knots 0 0 0 1 2 2 2
  spline S178 degree 2 poles (85.7802, 2.7019) (85.8957, 2.7019) (86.0385, 2.8103) (86.0385, 2.8984) knots 0 0 0 1 2 2 2
  spline S179 degree 2 poles (86.0385, 2.8984) (86.0385, 2.9775) (85.9544, 3.0717) (85.8754, 3.0929) knots 0 0 0 1 2 2 2
  spline S180 degree 2 poles (85.8754, 3.0929) (85.8227, 3.1071) (85.6698, 3.1436) (85.6191, 3.1588) knots 0 0 0 1 2 2 2
  spline S181 degree 2 poles (85.6191, 3.1588) (85.4905, 3.1983) (85.3709, 3.3573) (85.3709, 3.4738) knots 0 0 0 1 2 2 2
  spline S182 degree 2 poles (85.3709, 3.4738) (85.3709, 3.5478) (85.4307, 3.6896) (85.4844, 3.7392) knots 0 0 0 1 2 2 2
  spline S183 degree 2 poles (85.4844, 3.7392) (85.5442, 3.7939) (85.6961, 3.8527) (85.8106, 3.8527) knots 0 0 0 1 2 2 2
  spline S184 degree 2 poles (84.4431, 3.3614) (84.4431, 3.5984) (84.671, 3.8567) (84.8614, 3.8567) knots 0 0 0 1 2 2 2
  spline S185 degree 2 poles (84.8614, 3.8567) (85.0569, 3.8567) (85.2808, 3.5903) (85.2808, 3.3614) knots 0 0 0 1 2 2 2
  spline S186 degree 2 poles (85.2808, 3.3614) (85.2808, 3.1264) (85.0498, 2.866) (84.8614, 2.866) knots 0 0 0 1 2 2 2
  spline S187 degree 2 poles (84.8614, 2.866) (84.671, 2.866) (84.4431, 3.1254) (84.4431, 3.3614) knots 0 0 0 1 2 2 2
  spline S188 degree 2 poles (84.6062, 3.3614) (84.6062, 3.179) (84.7389, 3.0018) (84.8614, 3.0018) knots 0 0 0 1 2 2 2
  spline S189 degree 2 poles (84.8614, 3.0018) (84.984, 3.0018) (85.1177, 3.179) (85.1177, 3.3614) knots 0 0 0 1 2 2 2
  spline S190 degree 2 poles (85.1177, 3.3614) (85.1177, 3.5386) (84.984, 3.721) (84.8614, 3.721) knots 0 0 0 1 2 2 2
  spline S191 degree 2 poles (84.8614, 3.721) (84.7399, 3.721) (84.6062, 3.5417) (84.6062, 3.3614) knots 0 0 0 1 2 2 2
  spline S192 degree 2 poles (83.4949, 3.3462) (83.4949, 3.5761) (83.7178, 3.8567) (83.8859, 3.8567) knots 0 0 0 1 2 2 2
  spline S193 degree 2 poles (83.8859, 3.8567) (83.9619, 3.8567) (84.0703, 3.8192) (84.123, 3.7868) knots 0 0 0 1 2 2 2
  line L182 (84.123, 3.7868) -> (84.1331, 3.8304)
  line L183 (84.1331, 3.8304) -> (84.281, 3.8304)
  line L184 (84.281, 3.8304) -> (84.281, 2.5247)
  line L185 (84.281, 2.5247) -> (84.123, 2.5247)
  line L186 (84.123, 2.5247) -> (84.123, 2.9906)
  spline S194 degree 2 poles (84.123, 2.9906) (84.0632, 2.9369) (83.9244, 2.866) (83.8363, 2.866) knots 0 0 0 1 2 2 2
  spline S195 degree 2 poles (83.8363, 2.866) (83.6773, 2.866) (83.4949, 3.1203) (83.4949, 3.3462) knots 0 0 0 1 2 2 2
  spline S196 degree 2 poles (83.658, 3.3583) (83.658, 3.1902) (83.7603, 3.016) (83.8738, 3.016) knots 0 0 0 1 2 2 2
  spline S197 degree 2 poles (83.8738, 3.016) (83.9376, 3.016) (84.0693, 3.0767) (84.123, 3.1233) knots 0 0 0 1 2 2 2
  line L187 (84.123, 3.1233) -> (84.123, 3.6612)
  spline S198 degree 2 poles (84.123, 3.6612) (84.0632, 3.6906) (83.971, 3.7149) (83.9163, 3.7149) knots 0 0 0 1 2 2 2
  spline S199 degree 2 poles (83.9163, 3.7149) (83.7958, 3.7149) (83.658, 3.5437) (83.658, 3.3583) knots 0 0 0 1 2 2 2
  spline S200 degree 2 poles (82.9581, 3.8516) (83.0553, 3.8516) (83.2164, 3.7919) (83.2741, 3.7311) knots 0 0 0 1 2 2 2
  spline S201 degree 2 poles (83.2741, 3.7311) (83.3318, 3.6713) (83.3957, 3.487) (83.3957, 3.3634) knots 0 0 0 1 2 2 2
  spline S202 degree 2 poles (83.3957, 3.3634) (83.3957, 3.2398) (83.3298, 3.0595) (83.2741, 2.9987) knots 0 0 0 1 2 2 2
  spline S203 degree 2 poles (83.2741, 2.9987) (83.2184, 2.9369) (83.0533, 2.8711) (82.9581, 2.8711) knots 0 0 0 1 2 2 2
  spline S204 degree 2 poles (82.9581, 2.8711) (82.8811, 2.8711) (82.7372, 2.9147) (82.6815, 2.943) knots 0 0 0 1 2 2 2
  line L188 (82.6815, 2.943) -> (82.6815, 3.1203)
  line L189 (82.6815, 3.1203) -> (82.6906, 3.1203)
  spline S205 degree 2 poles (82.6906, 3.1203) (82.7079, 3.1061) (82.7605, 3.0696) (82.798, 3.0504) knots 0 0 0 1 2 2 2
  spline S206 degree 2 poles (82.798, 3.0504) (82.8314, 3.0342) (82.9206, 3.0089) (82.9611, 3.0089) knots 0 0 0 1 2 2 2
  spline S207 degree 2 poles (82.9611, 3.0089) (83.0837, 3.0089) (83.2326, 3.1942) (83.2326, 3.3634) knots 0 0 0 1 2 2 2
  spline S208 degree 2 poles (83.2326, 3.3634) (83.2326, 3.5285) (83.0887, 3.7139) (82.9611, 3.7139) knots 0 0 0 1 2 2 2
  spline S209 degree 2 poles (82.9611, 3.7139) (82.8841, 3.7139) (82.7443, 3.6501) (82.6906, 3.6004) knots 0 0 0 1 2 2 2
  line L190 (82.6906, 3.6004) -> (82.6815, 3.6004)
  line L191 (82.6815, 3.6004) -> (82.6815, 3.7777)
  spline S210 degree 2 poles (82.6815, 3.7777) (82.7048, 3.7888) (82.7757, 3.8202) (82.8041, 3.8273) knots 0 0 0 1 2 2 2
  spline S211 degree 2 poles (82.8041, 3.8273) (82.8446, 3.8395) (82.9084, 3.8516) (82.9581, 3.8516) knots 0 0 0 1 2 2 2
  line L192 (82.7018, 2.4234) -> (82.8932, 2.7414)
  line L193 (82.8932, 2.7414) -> (83.0837, 2.7414)
  line L194 (83.0837, 2.7414) -> (83.2751, 2.4234)
  line L195 (83.2751, 2.4234) -> (83.1414, 2.4234)
  line L196 (83.1414, 2.4234) -> (82.9864, 2.6381)
  line L197 (82.9864, 2.6381) -> (82.8314, 2.4234)
  line L198 (82.8314, 2.4234) -> (82.7018, 2.4234)
  line L199 (81.8083, 3.8304) -> (81.9664, 3.8304)
  line L200 (81.9664, 3.8304) -> (81.9664, 3.7271)
  spline S212 degree 2 poles (81.9664, 3.7271) (82.0393, 3.7909) (82.17, 3.8567) (82.251, 3.8567) knots 0 0 0 1 2 2 2
  spline S213 degree 2 poles (82.251, 3.8567) (82.3118, 3.8567) (82.4202, 3.8162) (82.4597, 3.7726) knots 0 0 0 1 2 2 2
  spline S214 degree 2 poles (82.4597, 3.7726) (82.5002, 3.7291) (82.5448, 3.5964) (82.5448, 3.5012) knots 0 0 0 1 2 2 2
  line L201 (82.5448, 3.5012) -> (82.5448, 2.8924)
  line L202 (82.5448, 2.8924) -> (82.3868, 2.8924)
  line L203 (82.3868, 2.8924) -> (82.3868, 3.4272)
  spline S215 degree 2 poles (82.3868, 3.4272) (82.3868, 3.5022) (82.3756, 3.6004) (82.3564, 3.6369) knots 0 0 0 1 2 2 2
  spline S216 degree 2 poles (82.3564, 3.6369) (82.3371, 3.6734) (82.2713, 3.7068) (82.2095, 3.7068) knots 0 0 0 1 2 2 2
  spline S217 degree 2 poles (82.2095, 3.7068) (82.1517, 3.7068) (82.0211, 3.641) (81.9664, 3.5933) knots 0 0 0 1 2 2 2
  line L204 (81.9664, 3.5933) -> (81.9664, 2.8924)
  line L205 (81.9664, 2.8924) -> (81.8083, 2.8924)
  line L206 (81.8083, 2.8924) -> (81.8083, 3.8304)
  line L207 (80.8025, 3.8304) -> (81.0101, 3.8304)
  line L208 (81.0101, 3.8304) -> (81.3586, 3.3776)
  line L209 (81.3586, 3.3776) -> (81.4214, 3.4384)
  line L210 (81.4214, 3.4384) -> (81.4214, 3.8304)
  line L211 (81.4214, 3.8304) -> (81.5794, 3.8304)
  line L212 (81.5794, 3.8304) -> (81.5794, 2.5247)
  line L213 (81.5794, 2.5247) -> (81.4214, 2.5247)
  line L214 (81.4214, 2.5247) -> (81.4214, 3.2884)
  line L215 (81.4214, 3.2884) -> (81.0506, 2.8924)
  line L216 (81.0506, 2.8924) -> (80.8541, 2.8924)
  line L217 (80.8541, 2.8924) -> (81.2391, 3.2844)
  line L218 (81.2391, 3.2844) -> (80.8025, 3.8304)
  point P0 (49.5, 15)
  dimension "d0" = 3
  dimension "d1" = 30
  dimension "d2" = 25
  dimension "d22" = 0.5
  dimension "d23" = 0.5
  constraints: 2 other
  measures "d22" distance between parallel lines of L0 L4
  measures "d23" distance between parallel lines of L1 L7
extrude "Vysunutí3" cut sketch "Náčrt3" against normal blind 0.2 contours L8 L9 L10 L11 L12 L13 L14 L15 L16 L17 | S0 S1 S2 S3 L18 L19 S4 S5 S6 L20 L21 S7 S8 | S13 S14 S15 S16 | S21 L23 L24 S22 S23 S24 S25 S26 S27 S28 S29 L25 L26 S30 S31 S32 S33 S34 S35 S36 | L27 L28 S37 S38 S39 L29 L30 L31 S40 S41 S42 L32 L33 L34 | L35 S43 S44 S45 S46 L36 L37 L38 S47 S48 S49 L39 L40 L41 L42 L43 S50 S51 S52 S53 S54 L44 L45 | S55 S56 S57 S58 L46 L47 S59 S60 S61 L48 L49 S62 S63 | S68 S69 S70 S71 S72 L51 L52 S73 S74 S75 S76 S77 L53 L54 S78 S79 | L55 L56 L57 L58 | L59 L60 L61 L62 L63 L64 L65 L66 L67 L68 L69 L70 L71 | L72 L73 L74 L75 L76 L77 L78 L79 L80 L81 L82 L83 | L84 L85 L86 L87 L88 L89 S80 L90 L91 L92 L93 | L94 L95 L96 L97 L98 L99 L100 L101 L102 L103 L104 L105 L106 | S81 S82 S83 S84 S85 S86 L107 S87 S88 S89 L108 L109 S90 S91 S92 L110 L111 L112 | L114 L115 S97 S98 S99 S100 S101 S102 S103 L116 L117 L118 | S108 S109 S110 S111 L120 L121 S112 S113 S114 L122 L123 S115 S116 | S121 S122 L125 L126 L127 L128 L129 S123 S124 | L131 L132 L133 L134 L135 L136 L137 L138 | L139 L140 L141 L142 L143 L144 L145 | S129 S130 S131 S132 S133 S134 L146 S135 S136 S137 L147 L148 S138 S139 S140 L149 L150 L151 | L153 L154 S145 S146 S147 S148 S149 S150 S151 L155 L156 L157 | L159 L160 L161 L162 | L163 L164 L165 L166 | L167 S156 S157 S158 S159 L168 L169 L170 S160 S161 S162 L171 L172 L173 L174 L175 S163 S164 S165 S166 S167 L176 L177 | S168 L178 L179 S169 S170 S171 S172 S173 S174 S175 S176 L180 L181 S177 S178 S179 S180 S181 S182 S183 | S184 S185 S186 S187 | S192 S193 L182 L183 L184 L185 L186 S194 S195 | S200 S201 S202 S203 S204 L188 L189 S205 S206 S207 S208 S209 L190 L191 S210 S211 | L192 L193 L194 L195 L196 L197 L198 | L199 L200 S212 S213 S214 L201 L202 L203 S215 S216 S217 L204 L205 L206 | L207 L208 L209 L210 L211 L212 L213 L214 L215 L216 L217 L218
chamfer "Zkosení1" distance 0.5 angle 45 3 edges at (-36.5, 1.5, -8) (-1.5, 1.5, -8) (33.5, 1.5, -8)
